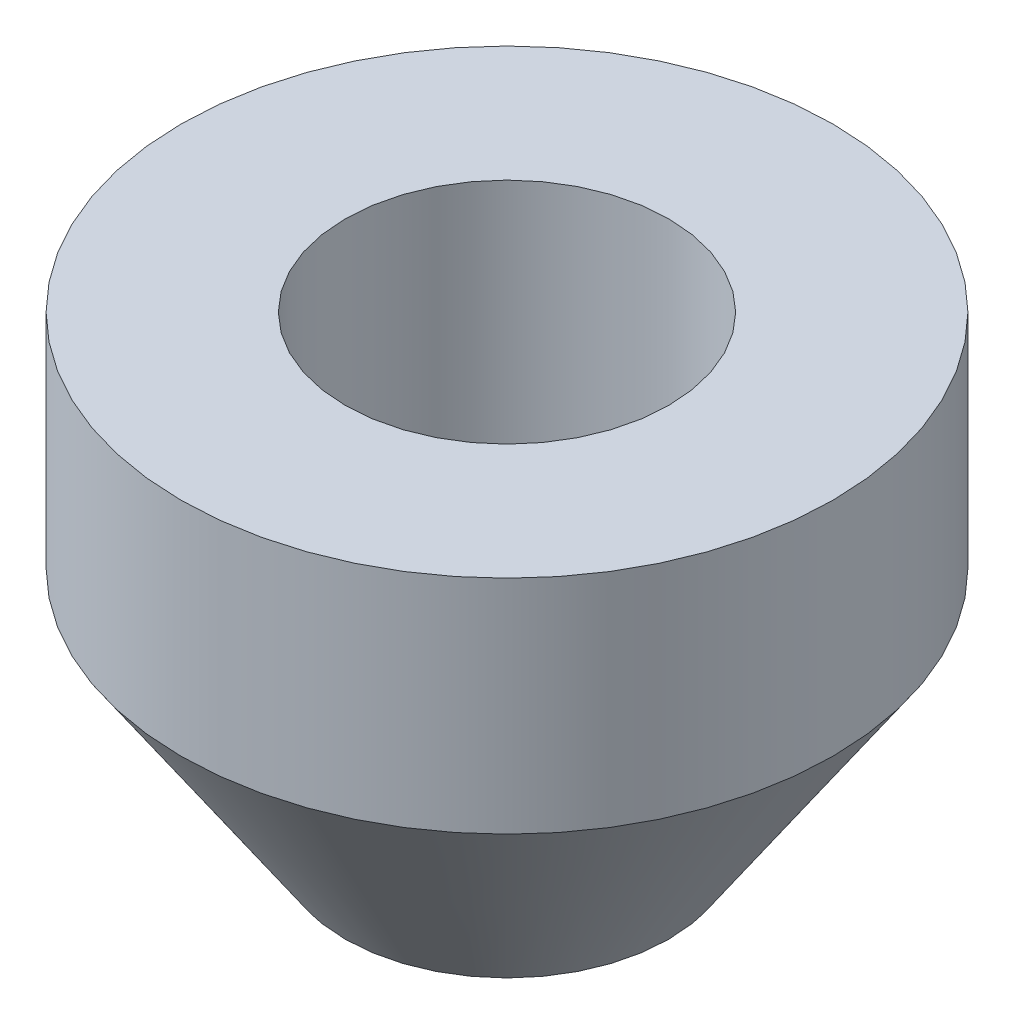
# Autodesk Inventor part: dickhead
Saved by Autodesk Inventor 2018 (Build 220112000, 112)
## iProperties
Created: 2018-12-04
Part Number: dickhead
Material: Generic
Document SubType Name: Modeling
Designer: Jerry
Density: 1 g/cm^3
Appearance: Default
Author: Jerry
Autodesk Inventor part; units mm, degrees
ref_plane "YZ Plane" through (0, 0, 0) normal (1, 0, 0) x (0, 1, 0)
ref_plane "XZ Plane" through (0, 0, 0) normal (0, 1, 0) x (-1, 0, 0)
ref_plane "XY Plane" through (0, 0, 0) normal (0, 0, 1) x (1, 0, 0)
sketch "Sketch1" plane through (0, 0, 0) normal (0, 0, 1) x (1, 0, 0)
  line L0 (3, 0) -> (3, -6.1892)
  line L1 (3, -6.1892) -> (0, -6.1892)
  line L2 (0, -6.1892) -> (0, -8.577)
  line L3 (0, -8.577) -> (3, -8.577)
  line L4 (3, -8.577) -> (6.0464, -4.1129)
  line L5 (6.0464, -4.1129) -> (6.0464, 0)
  line L6 (6.0464, 0) -> (3, 0)
  point P0 (0, 0)
  constraints: 14 end point, 4 perpendicular, 2 vertical, 1 point on line
revolve "Revolution1" add sketch "Sketch1" angle 360 about axis through (0, -6.1892, 0) along (0, -1, 0)
thread "Thread1" size "M6x1" class "6H" standard "ANSI Metric M Profile" full length
body "Solid1"
